Autodesk Fusion 360 part; units mm, degrees
(part 2 of 2)
equation "b_ = 5 mm" comment "added by script"
named bodies: "b  stock body", "b top  final body", "b top circles circle body", "b top circles circle body (1)", "b top circles circle body (2)", "b top circles circle body (3)", "b top circles circle body (4)", "b top circles circle body (5)", "b top circles circle body (6)", "b top circles circle body (7)", "b top circles circle body (8)", "b top circles circle body (9)", "b top circles circle body (10)", "b top circles circle body (11)", "b top circles circle body (12)", "b top circles circle body (13)", "b top circles circle body (14)", "b top circles circle body (15)", "b top circles circle body (16)", "b top circles circle body (17)", "b top circles circle body (18)", "b top circles circle body (19)", "b top circles circle body (20)", "b top circles circle body (21)", "b top circles circle body (22)", "b top circles circle body (23)", "b top circles circle body (24)", "b top circles circle body (25)", "b top circles circle body (26)", "b top circles circle body (27)", "b bottom  final body", "b bottom circles circle body", "b bottom circles circle body (1)", "b bottom circles circle body (2)", "b bottom circles circle body (3)", "b bottom circles circle body (4)", "b bottom circles circle body (5)", "b bottom circles circle body (6)", "b bottom circles circle body (7)", "b bottom circles circle body (8)", "b bottom circles circle body (9)", "b bottom circles circle body (10)", "b bottom circles circle body (11)", "b bottom circles circle body (12)", "b bottom circles circle body (13)", "b bottom circles circle body (14)", "b bottom circles circle body (15)", "b bottom circles circle body (16)", "b bottom circles circle body (17)", "b bottom circles circle body (18)", "b bottom circles circle body (19)", "b bottom circles circle body (20)", "b bottom circles circle body (21)", "b bottom circles circle body (22)", "b bottom circles circle body (23)", "b bottom circles circle body (24)", "b bottom circles circle body (25)", "b bottom circles circle body (26)", "b bottom circles circle body (27)", "b left  final body", "b left circles circle body", "b left circles circle body (1)", "b left circles circle body (2)", "b left circles circle body (3)", "b left circles circle body (4)", "b left circles circle body (5)", "b left circles circle body (6)", "b left circles circle body (7)", "b left circles circle body (8)", "b left circles circle body (9)", "b left circles circle body (10)", "b left circles circle body (11)", "b left circles circle body (12)", "b left circles circle body (13)", "b left circles circle body (14)", "b left circles circle body (15)", "b left circles circle body (16)", "b left circles circle body (17)", "b left circles circle body (18)", "b left circles circle body (19)", "b right  final body", "b right circles circle body", "b right circles circle body (1)", "b right circles circle body (2)", "b right circles circle body (3)", "b right circles circle body (4)", "b right circles circle body (5)", "b right circles circle body (6)", "b right circles circle body (7)", "b right circles circle body (8)", "b right circles circle body (9)", "b right circles circle body (10)", "b right circles circle body (11)", "b right circles circle body (12)", "b right circles circle body (13)", "b right circles circle body (14)", "b right circles circle body (15)", "b right circles circle body (16)", "b right circles circle body (17)", "b right circles circle body (18)", "b right circles circle body (19)", "b front  final body", "b front circles circle body", "b front circles circle body (1)", "b front circles circle body (2)", "b front circles circle body (3)", "b front circles circle body (4)", "b front circles circle body (5)", "b front circles circle body (6)", "b front circles circle body (7)", "b front circles circle body (8)", "b front circles circle body (9)", "b front circles circle body (10)", "b front circles circle body (11)", "b front circles circle body (12)", "b front circles circle body (13)", "b front circles circle body (14)", "b front circles circle body (15)", "b front circles circle body (16)", "b front circles circle body (17)", "b front circles circle body (18)", "b front circles circle body (19)", "b front circles circle body (20)", "b front circles circle body (21)", "b front circles circle body (22)", "b front circles circle body (23)", "b back  final body", "b back circles circle body", "b back circles circle body (1)", "b back circles circle body (2)", "b back circles circle body (3)", "b back circles circle body (4)", "b back circles circle body (5)", "b back circles circle body (6)", "b back circles circle body (7)", "b back circles circle body (8)", "b back circles circle body (9)", "b back circles circle body (10)", "b back circles circle body (11)", "b back circles circle body (12)", "b back circles circle body (13)", "b back circles circle body (14)", "b back circles circle body (15)", "b back circles circle body (16)", "b back circles circle body (17)", "b back circles circle body (18)", "b back circles circle body (19)", "b back circles circle body (20)", "b back circles circle body (21)", "b back circles circle body (22)", "b back circles circle body (23)"
